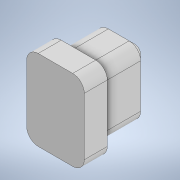
# Autodesk Inventor part: Button_Extender
Saved by Autodesk Inventor 2021 (Build 250183000, 183)
## iProperties
Created: 2025-03-05
Part Number: Button_Extender
Material: Generic
Document SubType Name: Modeling
Designer: Lukas
Density: 1 g/cm^3
Appearance: Default
Author: Lukas
Autodesk Inventor part; units mm, degrees
ref_plane "YZ Plane" through (0, 0, 0) normal (1, 0, 0) x (0, 1, 0)
ref_plane "XZ Plane" through (0, 0, 0) normal (0, 1, 0) x (-1, 0, 0)
ref_plane "XY Plane" through (0, 0, 0) normal (0, 0, 1) x (1, 0, 0)
sketch "Sketch1" plane through (0, 0, 0) normal (0, 0, 1) x (1, 0, 0)
  line L0 (-0.9, 2.9) -> (0.9, 2.9)
  line L1 (1.9, 1.9) -> (1.9, -1.9)
  line L2 (0.9, -2.9) -> (-0.9, -2.9)
  line L3 (-1.9, -1.9) -> (-1.9, 1.9)
  arc A0 (1.9, 1.9) -> (0.9, 2.9) centre (0.9, 1.9) ccw
  arc A1 (0.9, -2.9) -> (1.9, -1.9) centre (0.9, -1.9) ccw
  arc A2 (-1.9, -1.9) -> (-0.9, -2.9) centre (-0.9, -1.9) ccw
  arc A3 (-0.9, 2.9) -> (-1.9, 1.9) centre (-0.9, 1.9) ccw
  point P0 (0, 0)
  point P1 (0, 2.9)
  point P2 (-1.9, 0)
  dimension "d1" = 3.8
  dimension "d2" = 5.8
  dimension "d3" = 1
  constraints: 8 end point, 8 point on circle, 8 tangent, 4 centre point, 3 equal radius, 2 midpoint, 2 parallel, 1 horizontal, 1 horizontal alignment, 1 perpendicular, 1 vertical alignment
  measures "d1" distance between parallel lines of L1 L3
  measures "d2" distance between parallel lines of L2 L0
  measures "d3" radius of A0
extrude "Extrusion1" add sketch "Sketch1" along normal blind 4
sketch "Sketch2" plane through (0, 0, 4) normal (0, 0, 1) x (1, 0, 0)
  line L0 (-1.5, 3.5) -> (1.5, 3.5)
  line L1 (2.5, 2.5) -> (2.5, -2.5)
  line L2 (1.5, -3.5) -> (-1.5, -3.5)
  line L3 (-2.5, -2.5) -> (-2.5, 2.5)
  arc A0 (2.5, 2.5) -> (1.5, 3.5) centre (1.5, 2.5) ccw
  arc A1 (-2.5, -2.5) -> (-1.5, -3.5) centre (-1.5, -2.5) ccw
  arc A2 (1.5, -3.5) -> (2.5, -2.5) centre (1.5, -2.5) ccw
  arc A3 (-1.5, 3.5) -> (-2.5, 2.5) centre (-1.5, 2.5) ccw
  point P0 (0, 0)
  point P1 (-2.5, 3.5)
  point P2 (2.5, -3.5)
  point P3 (2.5, 3.5)
  point P4 (0, 3.5)
  point P5 (2.5, 0)
  dimension "d6" = 5
  dimension "d7" = 7
  dimension "d9" = 1
  constraints: 8 end point, 8 point on circle, 8 point on line, 8 tangent, 4 centre point, 3 equal radius, 2 midpoint, 2 parallel, 1 horizontal, 1 horizontal alignment, 1 perpendicular, 1 vertical alignment
  measures "d6" distance of point (-2.5, 3.5) point (2.5, 3.5)
  measures "d7" distance of point (2.5, 3.5) point (2.5, -3.5)
  measures "d9" radius of A3
extrude "Extrusion2" add sketch "Sketch2" along normal blind 2
chamfer "Chamfer1" distance 0.5 angle 45 8 edges at (-1.9, 0, 0) (-1.6071, -2.6071, 0) (0, -2.9, 0) (1.6071, -2.6071, 0) (1.9, 0, 0) (1.6071, 2.6071, 0) (0, 2.9, 0) (-1.6071, 2.6071, 0)
body "Solid1"
